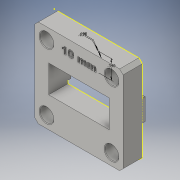
# Autodesk Inventor part: Cage Plate Slit 10mm
Saved by Autodesk Inventor 2016 (Build 200138000, 138)
## iProperties
Created: 2015-08-27
Part Number: Cage Plate Slit 10mm
Material: Generic
Document SubType Name: Modeling
Designer: kthorn
Density: 1 g/cm^3
Appearance: Default
Author: kthorn
Autodesk Inventor part; units mm, degrees
ref_plane "YZ Plane" through (0, 0, 0) normal (1, 0, 0) x (0, 1, 0)
ref_plane "XZ Plane" through (0, 0, 0) normal (0, 1, 0) x (-1, 0, 0)
ref_plane "XY Plane" through (0, 0, 0) normal (0, 0, 1) x (1, 0, 0)
sketch "Sketch1" plane through (0, 0, 0) normal (0, 0, 1) x (1, 0, 0)
  line L0 (1.5875, 0) -> (39.0525, 0)
  line L1 (40.64, -1.5875) -> (40.64, -39.0525)
  line L2 (39.0525, -40.64) -> (1.5875, -40.64)
  line L3 (0, -39.0525) -> (0, -1.5875)
  line L4 (5.3213, -5.3213) -> (35.3187, -5.3213) construction
  line L5 (35.3187, -5.3213) -> (35.3187, -35.3187) construction
  line L6 (35.3187, -35.3187) -> (5.3213, -35.3187) construction
  line L7 (5.3213, -35.3187) -> (5.3213, -5.3213) construction
  line L8 (35.3187, -5.3213) -> (40.64, 0) construction
  line L9 (5.3213, -35.3187) -> (0, -40.64) construction
  line L10 (5.3213, -5.3213) -> (0, 0) construction
  circle A0 centre (5.3213, -5.3213) radius 3.175
  circle A1 centre (35.3187, -5.3213) radius 3.175
  circle A2 centre (35.3187, -35.3187) radius 3.175
  circle A3 centre (5.3213, -35.3187) radius 3.175
  line L11 (1.5875, 0) -> (0, -1.5875)
  line L12 (0, -39.0525) -> (1.5875, -40.64)
  line L13 (39.0525, 0) -> (40.64, -1.5875)
  line L14 (40.64, -39.0525) -> (39.0525, -40.64)
  point P0 (40.64, -40.64)
  point P1 (40.64, -40.64)
  dimension "d0" = 40.64
  dimension "d1" = 29.9974
  dimension "d2" = 6.35
  dimension "d3" = 1.5875
  dimension "d4" = 1.5875
  dimension "d5" = 1.5875
  dimension "d6" = 1.5875
  dimension "d7" = 1.5875
  dimension "d8" = 1.5875
  dimension "d11" = 1.5875
  dimension "d12" = 1.5875
  constraints: 30 end point, 10 point on line, 6 perpendicular, 5 coincident, 4 centre point, 4 parallel, 3 equal radius, 2 horizontal
  measures "d0" distance of L10.end L8.end
  measures "d1" distance of L4.start L4.end
  measures "d2" diameter of A0
  measures "d3" distance of L0.start L10.end
  measures "d4" distance of L3.end L10.end
  measures "d5" distance of L3.start L9.end
  measures "d6" distance of L2.end L9.end
  measures "d7" distance of L0.end L8.end
  measures "d8" distance of L1.start L8.end
  measures "d11" distance of L1.end point (40.64, -40.64)
  measures "d12" distance of L2.start point (40.64, -40.64)
extrude "Extrusion1" add sketch "Sketch1" along normal blind 8.89
sketch "Sketch2" plane through (0, 0, 8.89) normal (0, 0, 1) x (1, 0, 0)
  circle A0 centre (5.3213, -35.3187) radius 3.175 projected
  circle A1 centre (35.3187, -35.3187) radius 3.175 projected
  circle A2 centre (35.3187, -5.3213) radius 3.175 projected
  circle A3 centre (5.3213, -5.3213) radius 3.175 projected
  line L0 (1.5875, 0) -> (0, -1.5875) projected
  line L1 (0, -1.5875) -> (0, -39.0525) projected
  line L2 (0, -39.0525) -> (1.5875, -40.64) projected
  line L3 (1.5875, -40.64) -> (39.0525, -40.64) projected
  line L4 (39.0525, -40.64) -> (40.64, -39.0525) projected
  line L5 (40.64, -39.0525) -> (40.64, -1.5875) projected
  line L6 (40.64, -1.5875) -> (39.0525, 0) projected
  line L7 (39.0525, 0) -> (1.5875, 0) projected
  line L8 (6.35, -20.32) -> (0, -20.32) construction
  line L9 (0, -1.5875) -> (0, -39.0525) projected
  line L10 (34.29, -20.32) -> (40.64, -20.32) construction
  line L11 (40.64, -39.0525) -> (40.64, -1.5875) projected
  line L12 (6.35, -13.97) -> (34.29, -13.97)
  line L13 (34.29, -13.97) -> (34.29, -26.67)
  line L14 (34.29, -26.67) -> (6.35, -26.67)
  line L15 (6.35, -26.67) -> (6.35, -13.97)
  line L16 (34.29, -26.67) -> (40.64, -26.67) construction
  point P0 (0, 0)
  dimension "d17" = 12.7
  dimension "d18" = 27.94
  constraints: 14 end point, 4 midpoint, 2 horizontal, 2 parallel, 2 perpendicular, 1 collinear, 1 point on line
  measures "d17" distance of L12.end L13.end
  measures "d18" distance of L13.end L14.end
sketch "Sketch3" plane through (0, 0, 8.89) normal (0, 0, 1) x (1, 0, 0)
  line L0 (9.5396, -2.9704) -> (31.1004, -2.9704) construction
  line L1 (31.1004, -2.9704) -> (31.1004, -7.6722) construction
  line L2 (31.1004, -7.6722) -> (9.5396, -7.6722) construction
  line L3 (9.5396, -7.6722) -> (9.5396, -2.9704) construction
  line L4 (37.465, 0) -> (0, 0)
  line L5 (0, 0) -> (0, -8.89)
  line L6 (37.465, -8.89) -> (0, -8.89)
  line L7 (37.465, 0) -> (37.465, -8.89)
  circle A0 centre (35.3187, -5.3213) radius 3.175 construction
  line L8 (35.3187, -5.3213) -> (31.1004, -5.3213) construction
  circle A1 centre (5.3213, -5.3213) radius 3.175 construction
  line L9 (5.3213, -5.3213) -> (9.5396, -5.3213) construction
  line L10 (14.3642, -3.6788) -> (14.3642, -6.9088)
  line L11 (14.3642, -6.9088) -> (13.4719, -6.9088)
  line L12 (13.4719, -6.9088) -> (13.4719, -4.7911)
  spline S0 degree 2 poles (13.4719, -4.7911) (13.2549, -4.9561) (12.8516, -5.1578) (12.546, -5.2525) knots 0 0 0 1 2 2 2
  line L13 (12.546, -5.2525) -> (12.546, -4.5283)
  spline S1 degree 2 poles (12.546, -4.5283) (12.9952, -4.3847) (13.4933, -3.9783) (13.6339, -3.6788) knots 0 0 0 1 2 2 2
  line L14 (13.6339, -3.6788) -> (14.3642, -3.6788)
  spline S2 degree 2 poles (15.3268, -5.3075) (15.3268, -4.403) (15.9777, -3.6788) (16.6438, -3.6788) knots 0 0 0 1 2 2 2
  spline S3 degree 2 poles (16.6438, -3.6788) (16.9647, -3.6788) (17.3742, -3.8377) (17.6339, -4.0913) (17.7837, -4.3694) (17.8295, -4.5558) knots 0 0 0 1 2 3 4 4 4
  spline S4 degree 2 poles (17.8295, -4.5558) (17.9181, -4.9103) (17.9181, -5.2984) knots 0 0 0 1 1 1
  spline S5 degree 2 poles (17.9181, -5.2984) (17.9181, -6.1632) (17.3345, -6.9638) (16.6194, -6.9638) knots 0 0 0 1 2 2 2
  spline S6 degree 2 poles (16.6194, -6.9638) (16.2191, -6.9638) (15.7271, -6.7071) (15.5682, -6.4596) knots 0 0 0 1 2 2 2
  spline S7 degree 2 poles (15.5682, -6.4596) (15.4551, -6.2854) (15.3268, -5.6773) (15.3268, -5.3075) knots 0 0 0 1 2 2 2
  spline S8 degree 2 poles (16.2008, -5.3106) (16.2008, -5.9187) (16.4147, -6.3618) (16.6163, -6.3618) knots 0 0 0 1 2 2 2
  spline S9 degree 2 poles (16.6163, -6.3618) (16.7508, -6.3618) (16.9494, -6.1723) (17.0411, -5.7659) (17.0411, -5.3351) knots 0 0 0 1 2 3 3 3
  spline S10 degree 2 poles (17.0411, -5.3351) (17.0411, -4.7025) (16.8272, -4.2655) (16.6133, -4.2655) knots 0 0 0 1 2 2 2
  spline S11 degree 2 poles (16.6133, -4.2655) (16.3963, -4.2655) (16.2008, -4.7086) (16.2008, -5.3106) knots 0 0 0 1 2 2 2
  line L15 (19.8555, -4.6078) -> (20.6775, -4.6078)
  line L16 (20.6775, -4.6078) -> (20.6775, -4.9439)
  spline S12 degree 2 poles (20.6775, -4.9439) (20.8548, -4.7331) (21.2184, -4.5558) (21.4751, -4.5558) knots 0 0 0 1 2 2 2
  spline S13 degree 2 poles (21.4751, -4.5558) (21.7501, -4.5558) (22.071, -4.7514) (22.1718, -4.9439) knots 0 0 0 1 2 2 2
  spline S14 degree 2 poles (22.1718, -4.9439) (22.3796, -4.7178) (22.7219, -4.5558) (22.9725, -4.5558) knots 0 0 0 1 2 2 2
  spline S15 degree 2 poles (22.9725, -4.5558) (23.3422, -4.5558) (23.7578, -4.9959) (23.7578, -5.4634) knots 0 0 0 1 2 2 2
  line L17 (23.7578, -5.4634) -> (23.7578, -6.9088)
  line L18 (23.7578, -6.9088) -> (22.8747, -6.9088)
  line L19 (22.8747, -6.9088) -> (22.8747, -5.5979)
  spline S16 degree 2 poles (22.8747, -5.5979) (22.8747, -5.442) (22.8136, -5.3656) knots 0 0 0 1 1 1
  spline S17 degree 2 poles (22.8136, -5.3656) (22.7249, -5.2464) (22.5935, -5.2464) knots 0 0 0 1 1 1
  spline S18 degree 2 poles (22.5935, -5.2464) (22.4377, -5.2464) (22.2482, -5.4726) (22.2482, -5.7201) knots 0 0 0 1 2 2 2
  line L20 (22.2482, -5.7201) -> (22.2482, -6.9088)
  line L21 (22.2482, -6.9088) -> (21.3651, -6.9088)
  line L22 (21.3651, -6.9088) -> (21.3651, -5.6406)
  spline S19 degree 2 poles (21.3651, -5.6406) (21.3651, -5.4909) (21.3468, -5.4359) knots 0 0 0 1 1 1
  spline S20 degree 2 poles (21.3468, -5.4359) (21.3193, -5.3503) (21.1817, -5.2434) (21.087, -5.2434) knots 0 0 0 1 2 2 2
  spline S21 degree 2 poles (21.087, -5.2434) (20.9342, -5.2434) (20.7386, -5.4726) (20.7386, -5.7354) knots 0 0 0 1 2 2 2
  line L23 (20.7386, -5.7354) -> (20.7386, -6.9088)
  line L24 (20.7386, -6.9088) -> (19.8555, -6.9088)
  line L25 (19.8555, -6.9088) -> (19.8555, -4.6078)
  line L26 (24.2926, -4.6078) -> (25.1146, -4.6078)
  line L27 (25.1146, -4.6078) -> (25.1146, -4.9439)
  spline S22 degree 2 poles (25.1146, -4.9439) (25.2918, -4.7331) (25.6555, -4.5558) (25.9122, -4.5558) knots 0 0 0 1 2 2 2
  spline S23 degree 2 poles (25.9122, -4.5558) (26.1872, -4.5558) (26.508, -4.7514) (26.6089, -4.9439) knots 0 0 0 1 2 2 2
  spline S24 degree 2 poles (26.6089, -4.9439) (26.8167, -4.7178) (27.1589, -4.5558) (27.4095, -4.5558) knots 0 0 0 1 2 2 2
  spline S25 degree 2 poles (27.4095, -4.5558) (27.7793, -4.5558) (28.1949, -4.9959) (28.1949, -5.4634) knots 0 0 0 1 2 2 2
  line L28 (28.1949, -5.4634) -> (28.1949, -6.9088)
  line L29 (28.1949, -6.9088) -> (27.3117, -6.9088)
  line L30 (27.3117, -6.9088) -> (27.3117, -5.5979)
  spline S26 degree 2 poles (27.3117, -5.5979) (27.3117, -5.442) (27.2506, -5.3656) knots 0 0 0 1 1 1
  spline S27 degree 2 poles (27.2506, -5.3656) (27.162, -5.2464) (27.0306, -5.2464) knots 0 0 0 1 1 1
  spline S28 degree 2 poles (27.0306, -5.2464) (26.8747, -5.2464) (26.6853, -5.4726) (26.6853, -5.7201) knots 0 0 0 1 2 2 2
  line L31 (26.6853, -5.7201) -> (26.6853, -6.9088)
  line L32 (26.6853, -6.9088) -> (25.8021, -6.9088)
  line L33 (25.8021, -6.9088) -> (25.8021, -5.6406)
  spline S29 degree 2 poles (25.8021, -5.6406) (25.8021, -5.4909) (25.7838, -5.4359) knots 0 0 0 1 1 1
  spline S30 degree 2 poles (25.7838, -5.4359) (25.7563, -5.3503) (25.6188, -5.2434) (25.5241, -5.2434) knots 0 0 0 1 2 2 2
  spline S31 degree 2 poles (25.5241, -5.2434) (25.3713, -5.2434) (25.1757, -5.4726) (25.1757, -5.7354) knots 0 0 0 1 2 2 2
  line L34 (25.1757, -5.7354) -> (25.1757, -6.9088)
  line L35 (25.1757, -6.9088) -> (24.2926, -6.9088)
  line L36 (24.2926, -6.9088) -> (24.2926, -4.6078)
  point P0 (-1.5875, 0)
  constraints: 12 end point, 2 horizontal, 2 midpoint, 1 collinear, 2 other
extrude "Extrusion4" cut sketch "Sketch3" against normal blind 0.889 contours L10 L11 L12 S0 L13 S1 L14 | S2 S3 S4 S5 S6 S7 | L15 L16 S12 S13 S14 S15 L17 L18 L19 S16 S17 S18 L20 L21 L22 S19 S20 S21 L23 L24 L25 | L26 L27 S22 S23 S24 S25 L28 L29 L30 S26 S27 S28 L31 L32 L33 S29 S30 S31 L34 L35 L36
extrude "Extrusion8" cut sketch "Sketch2" against normal through all contours L12 L13 L14 L15
sketch "Sketch4" plane through (0, 0, 0) normal (0, 0, -1) x (-1, 0, 0)
  circle A0 centre (-5.3213, -35.3187) radius 3.175 projected
  circle A1 centre (-35.3187, -35.3187) radius 3.175 projected
  circle A2 centre (-35.3187, -5.3213) radius 3.175 projected
  circle A3 centre (-5.3213, -5.3213) radius 3.175 projected
  line L0 (-1.5875, 0) -> (0, -1.5875) projected
  line L1 (-39.0525, 0) -> (-1.5875, 0) projected
  line L2 (-40.64, -1.5875) -> (-39.0525, 0) projected
  line L3 (-40.64, -39.0525) -> (-40.64, -1.5875) projected
  line L4 (-39.0525, -40.64) -> (-40.64, -39.0525) projected
  line L5 (-1.5875, -40.64) -> (-39.0525, -40.64) projected
  line L6 (0, -39.0525) -> (-1.5875, -40.64) projected
  line L7 (0, -1.5875) -> (0, -39.0525) projected
  line L8 (0, -1.5875) -> (0, -39.0525) projected
  line L9 (-40.64, -25.32) -> (-34.29, -25.32)
  line L10 (-34.29, -25.32) -> (-34.29, -15.32)
  line L11 (-34.29, -15.32) -> (-40.64, -15.32)
  line L12 (-40.64, -15.32) -> (-40.64, -25.32)
  line L13 (-39.0525, 0) -> (-1.5875, 0) construction
  line L14 (-20.32, 0) -> (-20.32, -40.64) construction
  line L15 (-1.5875, -40.64) -> (-39.0525, -40.64) construction
  line L16 (0, -25.32) -> (-6.35, -25.32)
  line L17 (-6.35, -25.32) -> (-6.35, -15.32)
  line L18 (-6.35, -15.32) -> (0, -15.32)
  line L19 (0, -15.32) -> (0, -25.32)
  line L20 (-34.29, -26.67) -> (-34.29, -13.97) projected
  line L21 (-6.35, -13.97) -> (-6.35, -26.67) projected
  point P0 (0, 0)
  point P1 (-40.64, -20.32)
  point P2 (0, -20.32)
  point P3 (-34.29, -20.32)
  dimension "d45" = 10
  dimension "d48" = 27.94
  constraints: 18 end point, 6 midpoint, 5 symmetric about line, 2 parallel, 1 horizontal, 1 perpendicular
  measures "d45" distance of L9.end L10.end
  measures "d48" distance of L18.start L10.end
extrude "Extrusion5" add sketch "Sketch4" along normal blind 1.27 contours L7 L16 L17 L18 | L11 L10 L9 L3
sketch "Sketch5" plane through (0, 0, 0) normal (0, 0, -1) x (-1, 0, 0)
  line L0 (0, -1.5875) -> (0, -15.32) projected
  line L1 (-1.5875, 0) -> (0, -1.5875) projected
  line L2 (-39.0525, 0) -> (-1.5875, 0) projected
  line L3 (-40.64, -1.5875) -> (-39.0525, 0) projected
  line L4 (-40.64, -39.0525) -> (-40.64, -25.32) projected
  circle A0 centre (-35.3187, -5.3213) radius 3.175 projected
  circle A1 centre (-5.3213, -5.3213) radius 3.175 projected
  circle A2 centre (-35.3187, -35.3187) radius 3.175 projected
  circle A3 centre (-5.3213, -35.3187) radius 3.175 projected
  line L5 (-40.64, -39.0525) -> (-40.64, -25.32) projected
  line L6 (-39.0525, -40.64) -> (-40.64, -39.0525) projected
  line L7 (-1.5875, -40.64) -> (-39.0525, -40.64) projected
  line L8 (0, -39.0525) -> (-1.5875, -40.64) projected
  line L9 (0, -1.5875) -> (0, -15.32) projected
  line L10 (-20.32, -15.32) -> (-20.32, -6.684) construction
  circle A4 centre (-20.32, -6.684) radius 1.7145
  circle A5 centre (-20.32, -6.684) radius 2.413
  line L11 (0, -1.5875) -> (0, -39.0525) construction
  line L12 (-40.64, -39.0525) -> (-40.64, -1.5875) construction
  line L13 (-1.5875, 0) -> (0, -1.5875) projected
  line L14 (-39.0525, 0) -> (-1.5875, 0) projected
  line L15 (-40.64, -1.5875) -> (-39.0525, 0) projected
  line L16 (-39.0525, -40.64) -> (-40.64, -39.0525) projected
  line L17 (-1.5875, -40.64) -> (-39.0525, -40.64) projected
  line L18 (0, -39.0525) -> (-1.5875, -40.64) projected
  line L19 (-34.29, -25.32) -> (-40.64, -25.32) projected
  line L20 (0, -25.32) -> (0, -39.0525) projected
  line L21 (0, -25.32) -> (-6.35, -25.32) projected
  line L22 (-6.35, -25.32) -> (-6.35, -26.67) projected
  line L23 (-6.35, -26.67) -> (-34.29, -26.67) projected
  line L24 (-34.29, -26.67) -> (-34.29, -25.32) projected
  line L25 (-40.64, -15.32) -> (-34.29, -15.32) projected
  line L26 (-34.29, -15.32) -> (-34.29, -13.97) projected
  line L27 (-34.29, -13.97) -> (-6.35, -13.97) projected
  line L28 (-6.35, -13.97) -> (-6.35, -15.32) projected
  line L29 (-6.35, -15.32) -> (0, -15.32) projected
  line L30 (-40.64, -15.32) -> (-40.64, -1.5875) projected
  line L31 (-34.29, -25.32) -> (-40.64, -25.32) projected
  line L32 (0, -25.32) -> (0, -39.0525) projected
  line L33 (0, -25.32) -> (-6.35, -25.32) projected
  line L34 (-6.35, -25.32) -> (-6.35, -26.67) projected
  line L35 (-6.35, -26.67) -> (-34.29, -26.67) projected
  line L36 (-34.29, -26.67) -> (-34.29, -25.32) projected
  line L37 (-40.64, -15.32) -> (-34.29, -15.32) projected
  line L38 (-34.29, -15.32) -> (-34.29, -13.97) projected
  line L39 (-34.29, -13.97) -> (-6.35, -13.97) projected
  line L40 (-6.35, -13.97) -> (-6.35, -15.32) projected
  line L41 (-6.35, -15.32) -> (0, -15.32) projected
  line L42 (-40.64, -15.32) -> (-40.64, -1.5875) projected
  line L43 (-40.64, -15.32) -> (0, -15.32) construction
  line L44 (-40.64, -20.32) -> (0, -20.32) construction
  circle A6 centre (-20.32, -33.956) radius 1.7145
  circle A7 centre (-20.32, -33.956) radius 2.413
  point P0 (0, 0)
  point P1 (-20.32, -29.464)
  dimension "d36" = 8.636
  dimension "d37" = 3.429
  dimension "d38" = 4.826
  constraints: 6 end point, 4 centre point, 4 coincident, 3 midpoint, 3 symmetric about line, 1 perpendicular, 1 vertical, 2 other
  measures "d36" distance of L10.start L10.end
  measures "d37" diameter of A4
  measures "d38" diameter of A5
extrude "Extrusion6" cut sketch "Sketch5" against normal blind 4.318 contours A4 | A6
extrude "Extrusion7" cut sketch "Sketch5" against normal blind 0.508 contours A5 | A6 | A7
chamfer "Chamfer2" distance 0.254 angle 45 4 edges at (32.1437, -5.3213, 0) (32.1437, -35.3187, 0) (2.1463, -35.3187, 0) (2.1463, -5.3213, 0)
chamfer "Chamfer3" distance 0.254 angle 45 4 edges at (32.1437, -5.3213, 8.89) (2.1463, -5.3213, 8.89) (2.1463, -35.3187, 8.89) (32.1437, -35.3187, 8.89)
equation "\"d4\" = d3"
equation "\"d5\" = d3"
equation "\"d6\" = d5"
equation "\"d8\" = d7"
equation "\"d11\" = d9"
equation "\"d12\" = d11"
equation "\"d9\" = 1.5875"
body "Solid1"
